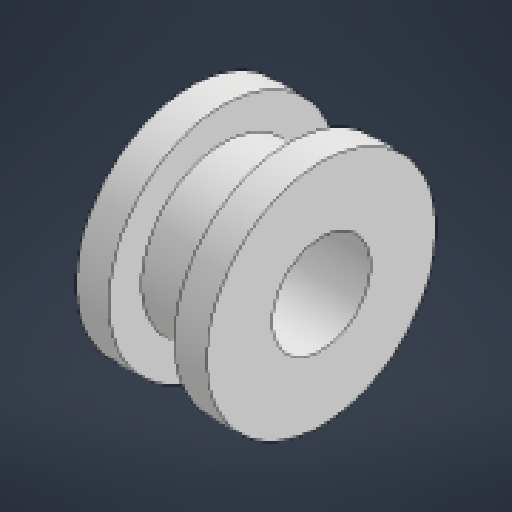
# Autodesk Inventor part: Pulley_MotorSide
Saved by Autodesk Inventor 2024.2 (Build 282272000, 272)
## iProperties
Created: 2023-12-22
Part Number: Pulley_MotorSide
Material: 一般
Document SubType Name: Modeling
Designer: Hanaoka
Density: 1 g/cm^3
Appearance: 既定
Author: Hanaoka
Autodesk Inventor part; units mm, degrees
ref_plane "YZ Plane" through (0, 0, 0) normal (1, 0, 0) x (0, 1, 0)
ref_plane "XZ Plane" through (0, 0, 0) normal (0, 1, 0) x (-1, 0, 0)
ref_plane "XY Plane" through (0, 0, 0) normal (0, 0, 1) x (1, 0, 0)
sketch "スケッチ1" plane through (0, 0, 0) normal (0, 1, 0) x (-1, 0, 0)
  line L0 (4, 0) -> (4, -3.5)
  line L1 (4, -3.5) -> (3, -3.5)
  line L2 (3, -3.5) -> (3, -2.5)
  line L3 (3, -2.5) -> (1, -2.5)
  line L4 (1, -2.5) -> (1, -3.5)
  line L5 (1, -3.5) -> (0, -3.5)
  line L6 (0, -3.5) -> (0, 0)
  line L7 (4, 0) -> (0, 0)
  line L8 (4, -1.5) -> (0, -1.5)
  dimension "d1" = 1
  dimension "d2" = 2
  dimension "d3" = 1.5
  dimension "d4" = 1
  dimension "d5" = 1
  constraints: 18 end point, 6 perpendicular, 3 equal length, 2 point on line, 2 vertical, 1 horizontal
  measures "d1" distance of L4.end L5.end
  measures "d2" distance of L2.end L3.end
  measures "d3" distance from line of L6.end L8
  measures "d4" distance between parallel lines of L8 L3
  measures "d5" distance of L1.end L2.end
revolve "回転1" add sketch "スケッチ1" angle 360 about axis through (-4, 0, 0) along (1, 0, 0) contours L0 L1 L2 L3 L4 L5 L6 L8
